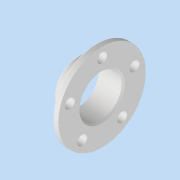
# Autodesk Inventor part: Gleit lager führung
Saved by Autodesk Inventor 2021 (Build 250183000, 183)
## iProperties
Created: 2024-03-15
Part Number: Gleit lager führung
Material: Generic
Document SubType Name: Modeling
Designer: Nokia
Density: 1 g/cm^3
Appearance: Default
Author: Nokia
Autodesk Inventor part; units mm, degrees
ref_plane "YZ Plane" through (0, 0, 0) normal (1, 0, 0) x (0, 1, 0)
ref_plane "XZ Plane" through (0, 0, 0) normal (0, 1, 0) x (-1, 0, 0)
ref_plane "XY Plane" through (0, 0, 0) normal (0, 0, 1) x (1, 0, 0)
sketch "Sketch1" plane through (0, 0, 0) normal (0, 0, 1) x (1, 0, 0)
  line L0 (0, 0) -> (0, 13)
  line L1 (0, 13) -> (-15, 13)
  line L2 (-15, 13) -> (-15, 15)
  line L3 (-15, 15) -> (-4, 15)
  line L4 (-4, 15) -> (-4, 27)
  line L5 (-4, 27) -> (0, 27)
  line L6 (0, 27) -> (0, 13)
  line L7 (0, 0) -> (-16.8305, 0)
  dimension "d0" = 13
  dimension "d1" = 15
  dimension "d2" = 2
  dimension "d4" = 12
  dimension "d6" = 4
  constraints: 16 end point, 6 perpendicular, 1 horizontal, 1 point on line, 1 vertical
  measures "d0" distance of L0.start L0.end
  measures "d1" distance of L0.end L1.end
  measures "d2" distance of L1.end L2.end
  measures "d4" distance of L3.end L4.end
  measures "d6" distance of L4.end L5.end
revolve "Revolution1" add sketch "Sketch1" angle 360 about axis through (0, 0, 0) along (-1, 0, 0)
sketch "Sketch2" plane through (0, 0, 0) normal (1, 0, 0) x (0, 0, -1)
  line L0 (0, 0) -> (0, 21)
  circle A0 centre (0, 21) radius 3
  circle A1 centre (-19.9722, 6.4894) radius 3
  circle A2 centre (-12.3435, -16.9894) radius 3
  circle A3 centre (12.3435, -16.9894) radius 3
  circle A4 centre (19.9722, 6.4894) radius 3
  dimension "d8" = 21
  dimension "d9" = 6
  dimension "d12" = 360
  constraints: 5 centre point, 2 end point, 1 coincident, 1 vertical, 11 other
  measures "d8" distance of L0.start L0.end
  measures "d9" diameter of A0
hole "Hole1" at (0, 6.4894, -19.9722) at (0, -16.9894, -12.3435) at (0, 21, 0) at (0, 6.4894, 19.9722) at (0, -16.9894, 12.3435) direction (-1, 0, 0) diameter 6 end through all
chamfer "Chamfer1" distance 1 angle 45 3 edges at (0, -13, 0) (-15, -15, 0) (-4, -27, 0)
body "Solid1"
